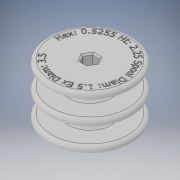
# Autodesk Inventor part: spool
Saved by Autodesk Inventor 2019.3 (Build 233278000, 278)
## iProperties
Created: 2019-02-25
Part Number: spool
Material: Generic
Document SubType Name: Modeling
Designer: steele
Density: 1 g/cm^3
Appearance: Default
Author: steele
Autodesk Inventor part; units mm, degrees
(part 1 of 2)
ref_plane "YZ Plane" through (0, 0, 0) normal (1, 0, 0) x (0, 1, 0)
ref_plane "XZ Plane" through (0, 0, 0) normal (0, 1, 0) x (-1, 0, 0)
ref_plane "XY Plane" through (0, 0, 0) normal (0, 0, 1) x (1, 0, 0)
sketch "Sketch1" plane through (0, 0, 0) normal (1, 0, 0) x (0, 1, 0)
  line L0 (0, 0) -> (0, -40.64)
  line L1 (3.81, -44.45) -> (3.81, -44.45)
  line L2 (7.62, -40.64) -> (7.62, -22.86)
  line L3 (11.43, -19.05) -> (20.955, -19.05)
  line L4 (24.765, -22.86) -> (24.765, -40.64)
  line L5 (28.575, -44.45) -> (28.575, -44.45)
  line L6 (32.385, -40.64) -> (32.385, -22.86)
  line L7 (36.195, -19.05) -> (45.72, -19.05)
  line L8 (49.53, -22.86) -> (49.53, -40.64)
  line L9 (53.34, -44.45) -> (53.34, -44.45)
  line L10 (57.15, -40.64) -> (57.15, 0)
  line L11 (0, 0) -> (57.15, 0)
  arc A0 (53.34, -44.45) -> (57.15, -40.64) centre (53.34, -40.64) ccw
  arc A1 (49.53, -40.64) -> (53.34, -44.45) centre (53.34, -40.64) ccw
  arc A2 (28.575, -44.45) -> (32.385, -40.64) centre (28.575, -40.64) ccw
  arc A3 (24.765, -40.64) -> (28.575, -44.45) centre (28.575, -40.64) ccw
  arc A4 (3.81, -44.45) -> (7.62, -40.64) centre (3.81, -40.64) ccw
  arc A5 (0, -40.64) -> (3.81, -44.45) centre (3.81, -40.64) ccw
  arc A6 (49.53, -22.86) -> (45.72, -19.05) centre (45.72, -22.86) ccw
  arc A7 (36.195, -19.05) -> (32.385, -22.86) centre (36.195, -22.86) ccw
  arc A8 (24.765, -22.86) -> (20.955, -19.05) centre (20.955, -22.86) ccw
  arc A9 (11.43, -19.05) -> (7.62, -22.86) centre (11.43, -22.86) ccw
  point P0 (49.53, -44.45)
  point P1 (57.15, -44.45)
  dimension "d0" = 57.15
  dimension "d1" = 7.62
  dimension "d2" = 19.05
  dimension "d3" = 44.45
  dimension "d4" = 3.81
  dimension "d5" = 3.81
  constraints: 24 end point, 20 point on circle, 20 tangent, 10 centre point, 8 equal radius, 6 perpendicular, 6 point on line, 5 collinear, 1 horizontal, 1 parallel, 1 vertical
  measures "d0" distance between parallel lines of L10 L0
  measures "d1" distance of point (49.53, -44.45) point (57.15, -44.45)
  measures "d2" distance between parallel lines of L3 L11
  measures "d3" distance between parallel lines of L1 L11
  measures "d4" radius of A0
  measures "d5" radius of A6
revolve "Revolution1" add sketch "Sketch1" angle 360 about axis through (0, 0, 0) along (0, 1, 0)
sketch "Sketch2" plane through (0, 57.15, 0) normal (0, 1, 0) x (1, 0, 0)
  line L0 (7.6623, 0) -> (3.8312, -6.6357)
  line L1 (3.8312, -6.6357) -> (-3.8312, -6.6357)
  line L2 (-3.8312, -6.6357) -> (-7.6623, 0)
  line L3 (-7.6623, 0) -> (-3.8312, 6.6357)
  line L4 (-3.8312, 6.6357) -> (3.8312, 6.6358)
  line L5 (3.8312, 6.6358) -> (7.6623, 0)
  point P0 (0, 0)
  point P1 (0, 0)
  dimension "d8" = 13.2715
  constraints: 12 end point, 1 coincident, 1 horizontal, 13 other
  measures "d8" distance between parallel lines of L1 L4
extrude "Extrusion1" cut sketch "Sketch2" against normal through all
sketch "Sketch4" plane through (0, 0, 0) normal (1, 0, 0) x (0, 1, 0)
  circle A0 centre (40.9575, 8.3858) radius 1.75
  circle A1 centre (16.1925, 8.3858) radius 1.75
  line L0 (7.62, 40.64) -> (7.62, -40.64) projected
  line L1 (49.53, 40.64) -> (49.53, -40.64) projected
  line L2 (57.15, 0) -> (0, 0) projected
  dimension "d17" = 8.5725
  dimension "d18" = 8.5725
  dimension "d19" = 3.5
  dimension "d20" = 8.3857
  dimension "d21" = 8.3857
  constraints: 2 centre point, 1 equal radius
  measures "d17" distance from line of A1.centre L0
  measures "d18" distance from line of A0.centre L1
  measures "d19" diameter of A0
  measures "d20" distance from line of A1.centre L2
  measures "d21" distance from line of A0.centre L2
extrude "Extrusion3" cut sketch "Sketch4" along normal through all both and the other way through all
chamfer "Chamfer2" distance 1.5875 angle 45 12 edges at (-5.7467, 57.15, -3.3179) (-5.7467, 57.15, 3.3179) (0, 57.15, 6.6357) (5.7467, 57.15, 3.3179) (0, 57.15, -6.6358) (0, 0, 6.6357) (5.7467, 0, 3.3179) (5.7467, 0, -3.3179) (0, 0, -6.6358) (-5.7467, 0, -3.3179) (-5.7467, 0, 3.3179) (5.7467, 57.15, -3.3179)
sketch "Sketch5" plane through (0, 57.15, 0) normal (0, 1, 0) x (1, 0, 0)
  circle A0 centre (0, 0) radius 33.3375
  line L0 (-33.0307, 5.0257) -> (-33.0993, 4.2184)
  line L1 (-33.0993, 4.2184) -> (-36.0724, 4.4709)
  line L2 (-36.0724, 4.4709) -> (-36.3098, 1.675)
  line L3 (-36.3098, 1.675) -> (-33.3367, 1.4226)
  line L4 (-33.3367, 1.4226) -> (-33.4052, 0.6153)
  line L5 (-33.4052, 0.6153) -> (-39.4794, 1.131)
  line L6 (-39.4794, 1.131) -> (-39.4108, 1.9383)
  line L7 (-39.4108, 1.9383) -> (-37.0284, 1.736)
  line L8 (-37.0284, 1.736) -> (-36.791, 4.5319)
  line L9 (-36.791, 4.5319) -> (-39.1734, 4.7342)
  line L10 (-39.1734, 4.7342) -> (-39.1049, 5.5414)
  line L11 (-39.1049, 5.5414) -> (-33.0307, 5.0257)
  spline S0 degree 2 poles (-32.2377, 8.0827) (-32.4935, 7.0163) (-33.9709, 6.1312) (-35.0757, 6.3963) knots 0 0 0 1 2 2 2
  spline S1 degree 2 poles (-35.0757, 6.3963) (-36.1614, 6.6568) (-37.1756, 8.1041) (-36.9555, 9.0216) knots 0 0 0 1 2 2 2
  spline S2 degree 2 poles (-36.9555, 9.0216) (-36.8563, 9.4348) (-36.4629, 10.016) (-36.1518, 10.1903) knots 0 0 0 1 2 2 2
  spline S3 degree 2 poles (-36.1518, 10.1903) (-35.8396, 10.3694) (-35.0435, 10.4477) (-34.5103, 10.3197) knots 0 0 0 1 2 2 2
  line L12 (-34.5103, 10.3197) -> (-34.102, 10.2218)
  line L13 (-34.102, 10.2218) -> (-34.8408, 7.1426)
  spline S4 degree 2 poles (-34.8408, 7.1426) (-34.0674, 6.957) (-33.0592, 7.5382) (-32.8933, 8.2299) knots 0 0 0 1 2 2 2
  spline S5 degree 2 poles (-32.8933, 8.2299) (-32.8345, 8.4749) (-32.8309, 8.9769) (-32.8712, 9.1898) knots 0 0 0 1 2 2 2
  spline S6 degree 2 poles (-32.8712, 9.1898) (-32.9189, 9.4147) (-33.0202, 9.7336) (-33.0751, 9.8433) knots 0 0 0 1 2 2 2
  line L14 (-33.0751, 9.8433) -> (-33.0648, 9.8865)
  line L15 (-33.0648, 9.8865) -> (-32.2481, 9.6906)
  spline S7 degree 2 poles (-32.2481, 9.6906) (-32.2264, 9.5482) (-32.1672, 9.1175) (-32.1609, 8.9534) knots 0 0 0 1 2 2 2
  spline S8 degree 2 poles (-32.1609, 8.9534) (-32.1503, 8.7222) (-32.1731, 8.3518) (-32.2377, 8.0827) knots 0 0 0 1 2 2 2
  spline S9 degree 2 poles (-34.8488, 9.6288) (-35.1538, 9.6918) (-35.6257, 9.6729) (-35.8034, 9.5885) knots 0 0 0 1 2 2 2
  spline S10 degree 2 poles (-35.8034, 9.5885) (-36.0026, 9.4992) (-36.2783, 9.1335) (-36.351, 8.8309) knots 0 0 0 1 2 2 2
  spline S11 degree 2 poles (-36.351, 8.8309) (-36.4224, 8.533) (-36.3449, 8.0725) (-36.2135, 7.8581) knots 0 0 0 1 2 2 2
  spline S12 degree 2 poles (-36.2135, 7.8581) (-36.0761, 7.6473) (-35.6901, 7.3718) (-35.4124, 7.2798) knots 0 0 0 1 2 2 2
  line L16 (-35.4124, 7.2798) -> (-34.8488, 9.6288)
  line L17 (-30.4327, 13.7615) -> (-30.7684, 12.8797)
  line L18 (-30.7684, 12.8797) -> (-32.7705, 12.4524)
  line L19 (-32.7705, 12.4524) -> (-31.5698, 10.7744)
  line L20 (-31.5698, 10.7744) -> (-31.8808, 9.9572)
  line L21 (-31.8808, 9.9572) -> (-33.4358, 12.2458)
  line L22 (-33.4358, 12.2458) -> (-36.1508, 11.5983)
  line L23 (-36.1508, 11.5983) -> (-35.8151, 12.4802)
  line L24 (-35.8151, 12.4802) -> (-33.8286, 12.9081)
  line L25 (-33.8286, 12.9081) -> (-35.019, 14.5716)
  line L26 (-35.019, 14.5716) -> (-34.708, 15.3888)
  line L27 (-34.708, 15.3888) -> (-33.1587, 13.1129)
  line L28 (-33.1587, 13.1129) -> (-30.4327, 13.7615)
  line L29 (-29.4968, 15.5425) -> (-29.94, 14.6706)
  line L30 (-29.94, 14.6706) -> (-30.9793, 15.1988)
  line L31 (-30.9793, 15.1988) -> (-30.536, 16.0708)
  line L32 (-30.536, 16.0708) -> (-29.4968, 15.5425)
  line L33 (-32.5353, 17.0871) -> (-32.9786, 16.2151)
  line L34 (-32.9786, 16.2151) -> (-34.0179, 16.7434)
  line L35 (-34.0179, 16.7434) -> (-33.5746, 17.6154)
  line L36 (-33.5746, 17.6154) -> (-32.5353, 17.0871)
  spline S13 degree 2 poles (-27.5071, 23.8971) (-26.2132, 22.8893) (-25.5869, 21.1931) (-26.1971, 20.4097) knots 0 0 0 1 2 2 2
  spline S14 degree 2 poles (-26.1971, 20.4097) (-26.8163, 19.6146) (-28.6316, 19.8324) (-29.8982, 20.819) knots 0 0 0 1 2 2 2
  spline S15 degree 2 poles (-29.8982, 20.819) (-31.2, 21.8328) (-31.8184, 23.523) (-31.2053, 24.3103) knots 0 0 0 1 2 2 2
  spline S16 degree 2 poles (-31.2053, 24.3103) (-30.5891, 25.1014) (-28.7621, 24.8745) (-27.5071, 23.8971) knots 0 0 0 1 2 2 2
  spline S17 degree 2 poles (-26.6852, 21.9295) (-26.8501, 22.2082) (-27.5221, 22.8568) (-28.0171, 23.2423) knots 0 0 0 1 2 2 2
  spline S18 degree 2 poles (-28.0171, 23.2423) (-28.5121, 23.6278) (-29.3016, 24.1175) (-29.623, 24.2113) knots 0 0 0 1 2 2 2
  spline S19 degree 2 poles (-29.623, 24.2113) (-29.9444, 24.3051) (-30.4619, 24.1633) (-30.6713, 23.8944) knots 0 0 0 1 2 2 2
  spline S20 degree 2 poles (-30.6713, 23.8944) (-30.8808, 23.6255) (-30.8976, 23.0813) (-30.7232, 22.7827) knots 0 0 0 1 2 2 2
  spline S21 degree 2 poles (-30.7232, 22.7827) (-30.5535, 22.494) (-29.8599, 21.841) (-29.3883, 21.4737) knots 0 0 0 1 2 2 2
  spline S22 degree 2 poles (-29.3883, 21.4737) (-28.8816, 21.0791) (-28.1549, 20.6133) (-27.8109, 20.5082) knots 0 0 0 1 2 2 2
  spline S23 degree 2 poles (-27.8109, 20.5082) (-27.4887, 20.4075) (-26.9496, 20.5449) (-26.731, 20.8255) knots 0 0 0 1 2 2 2
  spline S24 degree 2 poles (-26.731, 20.8255) (-26.5246, 21.0906) (-26.5078, 21.6347) (-26.6852, 21.9295) knots 0 0 0 1 2 2 2
  line L37 (-23.637, 23.5142) -> (-24.3167, 22.8108)
  line L38 (-24.3167, 22.8108) -> (-25.1551, 23.6209)
  line L39 (-25.1551, 23.6209) -> (-24.4754, 24.3243)
  line L40 (-24.4754, 24.3243) -> (-23.637, 23.5142)
  spline S25 degree 2 poles (-21.1932, 28.2583) (-20.9113, 27.9209) (-20.646, 27.1641) (-20.6658, 26.7871) knots 0 0 0 1 2 2 2
  spline S26 degree 2 poles (-20.6658, 26.7871) (-20.6856, 26.4101) (-21.0674, 25.6728) (-21.4313, 25.3688) knots 0 0 0 1 2 2 2
  spline S27 degree 2 poles (-21.4313, 25.3688) (-21.7649, 25.09) (-22.5405, 24.6932) (-22.8776, 24.6111) knots 0 0 0 1 2 2 2
  line L41 (-22.8776, 24.6111) -> (-23.4318, 25.2746)
  line L42 (-23.4318, 25.2746) -> (-23.3863, 25.3126)
  spline S28 degree 2 poles (-23.3863, 25.3126) (-23.2699, 25.3197) (-22.8868, 25.4081) (-22.6731, 25.4836) knots 0 0 0 1 2 2 2
  spline S29 degree 2 poles (-22.6731, 25.4836) (-22.4335, 25.5744) (-22.0662, 25.7589) (-21.8728, 25.9204) knots 0 0 0 1 2 2 2
  spline S30 degree 2 poles (-21.8728, 25.9204) (-21.6833, 26.0788) (-21.4409, 26.513) (-21.4356, 26.7685) knots 0 0 0 1 2 2 2
  spline S31 degree 2 poles (-21.4356, 26.7685) (-21.4352, 27.0069) (-21.6243, 27.4798) (-21.8333, 27.73) knots 0 0 0 1 2 2 2
  spline S32 degree 2 poles (-21.8333, 27.73) (-22.0423, 27.9803) (-22.4449, 28.1847) (-22.6624, 28.1832) knots 0 0 0 1 2 2 2
  spline S33 degree 2 poles (-22.6624, 28.1832) (-22.8933, 28.1899) (-23.3699, 27.959) (-23.6088, 27.7595) knots 0 0 0 1 2 2 2
  spline S34 degree 2 poles (-23.6088, 27.7595) (-23.8666, 27.5441) (-24.3119, 27.037) (-24.4388, 26.873) knots 0 0 0 1 2 2 2
  line L43 (-24.4388, 26.873) -> (-26.4531, 29.2842)
  line L44 (-26.4531, 29.2842) -> (-23.8865, 31.4283)
  line L45 (-23.8865, 31.4283) -> (-23.4273, 30.8786)
  line L46 (-23.4273, 30.8786) -> (-25.3911, 29.238)
  line L47 (-25.3911, 29.238) -> (-24.3491, 27.9907)
  spline S35 degree 2 poles (-24.3491, 27.9907) (-24.248, 28.1009) (-24.0377, 28.296) (-23.9467, 28.372) knots 0 0 0 1 2 2 2
  spline S36 degree 2 poles (-23.9467, 28.372) (-23.5865, 28.6729) (-22.9917, 28.9702) (-22.6185, 28.9859) knots 0 0 0 1 2 2 2
  spline S37 degree 2 poles (-22.6185, 28.9859) (-22.2416, 29.0047) (-21.5479, 28.683) (-21.1932, 28.2583) knots 0 0 0 1 2 2 2
  line L48 (-16.0539, 29.2803) -> (-19.2411, 27.2867)
  line L49 (-19.2411, 27.2867) -> (-19.6996, 28.0196)
  spline S38 degree 2 poles (-19.6996, 28.0196) (-19.5579, 28.5569) (-19.321, 29.5383) (-19.2295, 30.0442) knots 0 0 0 1 2 2 2
  spline S39 degree 2 poles (-19.2295, 30.0442) (-19.0451, 31.0627) (-19.1009, 32.1116) (-19.3603, 32.5262) knots 0 0 0 1 2 2 2
  spline S40 degree 2 poles (-19.3603, 32.5262) (-19.4965, 32.744) (-19.8349, 32.9868) (-20.0218, 33.0156) knots 0 0 0 1 2 2 2
  spline S41 degree 2 poles (-20.0218, 33.0156) (-20.2088, 33.0443) (-20.5926, 32.9499) (-20.7852, 32.8294) knots 0 0 0 1 2 2 2
  spline S42 degree 2 poles (-20.7852, 32.8294) (-20.9695, 32.7141) (-21.2888, 32.3862) (-21.416, 32.2076) knots 0 0 0 1 2 2 2
  spline S43 degree 2 poles (-21.416, 32.2076) (-21.5259, 32.0573) (-21.6934, 31.7195) (-21.7404, 31.6085) knots 0 0 0 1 2 2 2
  line L50 (-21.7404, 31.6085) -> (-21.7781, 31.5849)
  line L51 (-21.7781, 31.5849) -> (-22.2392, 32.322)
  spline S44 degree 2 poles (-22.2392, 32.322) (-22.0911, 32.5603) (-21.453, 33.2449) (-21.1096, 33.4598) knots 0 0 0 1 2 2 2
  spline S45 degree 2 poles (-21.1096, 33.4598) (-20.385, 33.913) (-19.0889, 33.6574) (-18.6803, 33.004) knots 0 0 0 1 2 2 2
  spline S46 degree 2 poles (-18.6803, 33.004) (-18.489, 32.6983) (-18.3118, 32.0982) (-18.3012, 31.8019) knots 0 0 0 1 2 2 2
  spline S47 degree 2 poles (-18.3012, 31.8019) (-18.2854, 31.4971) (-18.3721, 30.8252) (-18.4395, 30.4859) knots 0 0 0 1 2 2 2
  spline S48 degree 2 poles (-18.4395, 30.4859) (-18.5435, 29.9256) (-18.8667, 28.6629) (-18.9666, 28.2916) knots 0 0 0 1 2 2 2
  line L52 (-18.9666, 28.2916) -> (-16.4285, 29.8792)
  line L53 (-16.4285, 29.8792) -> (-16.0539, 29.2803)
  spline S49 degree 2 poles (-12.7562, 32.9388) (-12.5762, 32.5377) (-12.5255, 31.7374) (-12.6466, 31.3798) knots 0 0 0 1 2 2 2
  spline S50 degree 2 poles (-12.6466, 31.3798) (-12.7676, 31.0222) (-13.3347, 30.4157) (-13.7673, 30.2214) knots 0 0 0 1 2 2 2
  spline S51 degree 2 poles (-13.7673, 30.2214) (-14.1639, 30.0434) (-15.018, 29.8712) (-15.3646, 29.8834) knots 0 0 0 1 2 2 2
  line L54 (-15.3646, 29.8834) -> (-15.7187, 30.6721)
  line L55 (-15.7187, 30.6721) -> (-15.6646, 30.6964)
  spline S52 degree 2 poles (-15.6646, 30.6964) (-15.5506, 30.6717) (-15.1578, 30.6531) (-14.9317, 30.668) knots 0 0 0 1 2 2 2
  spline S53 degree 2 poles (-14.9317, 30.668) (-14.6764, 30.6906) (-14.273, 30.7688) (-14.0431, 30.872) knots 0 0 0 1 2 2 2
  spline S54 degree 2 poles (-14.0431, 30.872) (-13.8178, 30.9731) (-13.467, 31.3256) (-13.3926, 31.5701) knots 0 0 0 1 2 2 2
  spline S55 degree 2 poles (-13.3926, 31.5701) (-13.3278, 31.7996) (-13.3818, 32.306) (-13.5154, 32.6034) knots 0 0 0 1 2 2 2
  spline S56 degree 2 poles (-13.5154, 32.6034) (-13.6489, 32.9009) (-13.9811, 33.2066) (-14.191, 33.264) knots 0 0 0 1 2 2 2
  spline S57 degree 2 poles (-14.191, 33.264) (-14.4114, 33.3329) (-14.9327, 33.2397) (-15.2167, 33.1122) knots 0 0 0 1 2 2 2
  spline S58 degree 2 poles (-15.2167, 33.1122) (-15.5231, 32.9746) (-16.089, 32.6069) (-16.2556, 32.4834) knots 0 0 0 1 2 2 2
  line L56 (-16.2556, 32.4834) -> (-17.5423, 35.3496)
  line L57 (-17.5423, 35.3496) -> (-14.4913, 36.7193)
  line L58 (-14.4913, 36.7193) -> (-14.1979, 36.0658)
  line L59 (-14.1979, 36.0658) -> (-16.5324, 35.0179)
  line L60 (-16.5324, 35.0179) -> (-15.8668, 33.5351)
  spline S59 degree 2 poles (-15.8668, 33.5351) (-15.7397, 33.6139) (-15.4844, 33.7447) (-15.3762, 33.7933) knots 0 0 0 1 2 2 2
  spline S60 degree 2 poles (-15.3762, 33.7933) (-14.9481, 33.9855) (-14.2949, 34.1108) (-13.9315, 34.0249) knots 0 0 0 1 2 2 2
  spline S61 degree 2 poles (-13.9315, 34.0249) (-13.5635, 33.941) (-12.9828, 33.4436) (-12.7562, 32.9388) knots 0 0 0 1 2 2 2
  spline S62 degree 2 poles (-8.1381, 34.3723) (-8.0145, 33.9504) (-8.0737, 33.1506) (-8.2424, 32.8129) knots 0 0 0 1 2 2 2
  spline S63 degree 2 poles (-8.2424, 32.8129) (-8.4112, 32.4752) (-9.0557, 31.9518) (-9.5109, 31.8185) knots 0 0 0 1 2 2 2
  spline S64 degree 2 poles (-9.5109, 31.8185) (-9.928, 31.6963) (-10.7976, 31.6424) (-11.1393, 31.7018) knots 0 0 0 1 2 2 2
  line L61 (-11.1393, 31.7018) -> (-11.3824, 32.5315)
  line L62 (-11.3824, 32.5315) -> (-11.3255, 32.5481)
  spline S65 degree 2 poles (-11.3255, 32.5481) (-11.216, 32.5082) (-10.8294, 32.4361) (-10.6033, 32.4199) knots 0 0 0 1 2 2 2
  spline S66 degree 2 poles (-10.6033, 32.4199) (-10.3474, 32.4074) (-9.937, 32.4298) (-9.6952, 32.5006) knots 0 0 0 1 2 2 2
  spline S67 degree 2 poles (-9.6952, 32.5006) (-9.4582, 32.5701) (-9.0625, 32.8713) (-8.9555, 33.1034) knots 0 0 0 1 2 2 2
  spline S68 degree 2 poles (-8.9555, 33.1034) (-8.8599, 33.3218) (-8.8443, 33.8309) (-8.936, 34.1438) knots 0 0 0 1 2 2 2
  spline S69 degree 2 poles (-8.936, 34.1438) (-9.0276, 34.4567) (-9.3149, 34.8049) (-9.515, 34.8904) knots 0 0 0 1 2 2 2
  spline S70 degree 2 poles (-9.515, 34.8904) (-9.724, 34.9888) (-10.2531, 34.9676) (-10.5518, 34.8801) knots 0 0 0 1 2 2 2
  spline S71 degree 2 poles (-10.5518, 34.8801) (-10.8742, 34.7857) (-11.485, 34.4987) (-11.6669, 34.3991) knots 0 0 0 1 2 2 2
  line L63 (-11.6669, 34.3991) -> (-12.5501, 37.4142)
  line L64 (-12.5501, 37.4142) -> (-9.3406, 38.3544)
  line L65 (-9.3406, 38.3544) -> (-9.1392, 37.667)
  line L66 (-9.1392, 37.667) -> (-11.595, 36.9476)
  line L67 (-11.595, 36.9476) -> (-11.1381, 35.3879)
  spline S72 degree 2 poles (-11.1381, 35.3879) (-11.0014, 35.4485) (-10.7306, 35.5433) (-10.6168, 35.5766) knots 0 0 0 1 2 2 2
  spline S73 degree 2 poles (-10.6168, 35.5766) (-10.1665, 35.7085) (-9.5024, 35.7435) (-9.154, 35.6087) knots 0 0 0 1 2 2 2
  spline S74 degree 2 poles (-9.154, 35.6087) (-8.801, 35.4754) (-8.2936, 34.9033) (-8.1381, 34.3723) knots 0 0 0 1 2 2 2
  line L68 (0.4356, 33.408) -> (-0.3734, 33.3649)
  line L69 (-0.3734, 33.3649) -> (-0.5322, 36.3445)
  line L70 (-0.5322, 36.3445) -> (-3.3341, 36.1951)
  line L71 (-3.3341, 36.1951) -> (-3.1753, 33.2156)
  line L72 (-3.1753, 33.2156) -> (-3.9843, 33.1725)
  line L73 (-3.9843, 33.1725) -> (-4.3088, 39.2598)
  line L74 (-4.3088, 39.2598) -> (-3.4998, 39.3029)
  line L75 (-3.4998, 39.3029) -> (-3.3725, 36.9153)
  line L76 (-3.3725, 36.9153) -> (-0.5706, 37.0647)
  line L77 (-0.5706, 37.0647) -> (-0.6978, 39.4523)
  line L78 (-0.6978, 39.4523) -> (0.1112, 39.4954)
  line L79 (0.1112, 39.4954) -> (0.4356, 33.408)
  spline S75 degree 2 poles (2.9791, 33.1192) (2.3534, 33.1653) (1.7015, 33.9316) (1.7585, 34.7051) knots 0 0 0 1 2 2 2
  line L80 (1.7585, 34.7051) -> (1.9446, 37.2324)
  line L81 (1.9446, 37.2324) -> (1.4273, 37.2705)
  line L82 (1.4273, 37.2705) -> (1.4741, 37.9061)
  line L83 (1.4741, 37.9061) -> (1.9914, 37.868)
  line L84 (1.9914, 37.868) -> (2.0879, 39.1785)
  line L85 (2.0879, 39.1785) -> (2.8565, 39.1219)
  line L86 (2.8565, 39.1219) -> (2.76, 37.8114)
  line L87 (2.76, 37.8114) -> (4.1739, 37.7072)
  line L88 (4.1739, 37.7072) -> (4.1271, 37.0717)
  line L89 (4.1271, 37.0717) -> (2.7132, 37.1758)
  line L90 (2.7132, 37.1758) -> (2.5532, 35.0032)
  spline S76 degree 2 poles (2.5532, 35.0032) (2.5278, 34.6583) (2.5244, 34.2771) (2.5962, 34.1084) knots 0 0 0 1 2 2 2
  spline S77 degree 2 poles (2.5962, 34.1084) (2.6547, 33.9604) (2.9545, 33.7947) (3.2206, 33.7751) knots 0 0 0 1 2 2 2
  spline S78 degree 2 poles (3.2206, 33.7751) (3.4078, 33.7613) (3.7659, 33.8489) (3.8473, 33.8775) knots 0 0 0 1 2 2 2
  line L91 (3.8473, 33.8775) -> (3.8916, 33.8743)
  line L92 (3.8916, 33.8743) -> (3.8408, 33.1845)
  spline S79 degree 2 poles (3.8408, 33.1845) (3.6197, 33.1414) (3.1712, 33.1051) (2.9791, 33.1192) knots 0 0 0 1 2 2 2
  line L93 (6.3371, 36.1989) -> (5.3715, 36.3547)
  line L94 (5.3715, 36.3547) -> (5.5572, 37.5056)
  line L95 (5.5572, 37.5056) -> (6.5229, 37.3498)
  line L96 (6.5229, 37.3498) -> (6.3371, 36.1989)
  line L97 (5.7941, 32.8338) -> (4.8284, 32.9896)
  line L98 (4.8284, 32.9896) -> (5.0142, 34.1406)
  line L99 (5.0142, 34.1406) -> (5.9798, 33.9847)
  line L100 (5.9798, 33.9847) -> (5.7941, 32.8338)
  line L101 (13.2755, 30.6402) -> (9.7459, 31.9343)
  line L102 (9.7459, 31.9343) -> (10.0435, 32.746)
  spline S80 degree 2 poles (10.0435, 32.746) (10.5547, 32.9637) (11.4751, 33.3787) (11.9307, 33.6168) knots 0 0 0 1 2 2 2
  spline S81 degree 2 poles (11.9307, 33.6168) (12.8482, 34.0959) (13.6423, 34.7834) (13.8106, 35.2426) knots 0 0 0 1 2 2 2
  spline S82 degree 2 poles (13.8106, 35.2426) (13.8991, 35.4838) (13.8833, 35.9) (13.7913, 36.0653) knots 0 0 0 1 2 2 2
  spline S83 degree 2 poles (13.7913, 36.0653) (13.6993, 36.2305) (13.3893, 36.4757) (13.176, 36.5539) knots 0 0 0 1 2 2 2
  spline S84 degree 2 poles (13.176, 36.5539) (12.9719, 36.6288) (12.517, 36.6798) (12.298, 36.6706) knots 0 0 0 1 2 2 2
  spline S85 degree 2 poles (12.298, 36.6706) (12.1118, 36.6652) (11.7423, 36.5902) (11.6258, 36.5593) knots 0 0 0 1 2 2 2
  line L103 (11.6258, 36.5593) -> (11.584, 36.5746)
  line L104 (11.584, 36.5746) -> (11.8833, 37.3909)
  spline S86 degree 2 poles (11.8833, 37.3909) (12.1624, 37.4202) (13.0945, 37.3362) (13.4748, 37.1968) knots 0 0 0 1 2 2 2
  spline S87 degree 2 poles (13.4748, 37.1968) (14.2772, 36.9026) (14.8704, 35.7222) (14.6051, 34.9987) knots 0 0 0 1 2 2 2
  spline S88 degree 2 poles (14.6051, 34.9987) (14.481, 34.6601) (14.1158, 34.1521) (13.8883, 33.9619) knots 0 0 0 1 2 2 2
  spline S89 degree 2 poles (13.8883, 33.9619) (13.6573, 33.7624) (13.0735, 33.4188) (12.7642, 33.2638) knots 0 0 0 1 2 2 2
  spline S90 degree 2 poles (12.7642, 33.2638) (12.2578, 33.0022) (11.0625, 32.4829) (10.708, 32.334) knots 0 0 0 1 2 2 2
  line L105 (10.708, 32.334) -> (13.5187, 31.3035)
  line L106 (13.5187, 31.3035) -> (13.2755, 30.6402)
  line L107 (15.1742, 29.6878) -> (14.2969, 30.1203)
  line L108 (14.2969, 30.1203) -> (14.8124, 31.166)
  line L109 (14.8124, 31.166) -> (15.6897, 30.7335)
  line L110 (15.6897, 30.7335) -> (15.1742, 29.6878)
  line L111 (19.4562, 27.1389) -> (16.2802, 29.1503)
  line L112 (16.2802, 29.1503) -> (16.7427, 29.8807)
  spline S91 degree 2 poles (16.7427, 29.8807) (17.2885, 29.9853) (18.2757, 30.1962) (18.7714, 30.3325) knots 0 0 0 1 2 2 2
  spline S92 degree 2 poles (18.7714, 30.3325) (19.7695, 30.6068) (20.691, 31.1108) (20.9527, 31.524) knots 0 0 0 1 2 2 2
  spline S93 degree 2 poles (20.9527, 31.524) (21.0901, 31.741) (21.1628, 32.1511) (21.1078, 32.3321) knots 0 0 0 1 2 2 2
  spline S94 degree 2 poles (21.1078, 32.3321) (21.0528, 32.5131) (20.8017, 32.8183) (20.6098, 32.9399) knots 0 0 0 1 2 2 2
  spline S95 degree 2 poles (20.6098, 32.9399) (20.4261, 33.0562) (19.9924, 33.2022) (19.7763, 33.2396) knots 0 0 0 1 2 2 2
  spline S96 degree 2 poles (19.7763, 33.2396) (19.5932, 33.2737) (19.2162, 33.2786) (19.0958, 33.273) knots 0 0 0 1 2 2 2
  line L113 (19.0958, 33.273) -> (19.0582, 33.2968)
  line L114 (19.0582, 33.2968) -> (19.5234, 34.0313)
  spline S97 degree 2 poles (19.5234, 34.0313) (19.8023, 34.0009) (20.6956, 33.7217) (21.0378, 33.5049) knots 0 0 0 1 2 2 2
  spline S98 degree 2 poles (21.0378, 33.5049) (21.7598, 33.0477) (22.09, 31.7685) (21.6776, 31.1175) knots 0 0 0 1 2 2 2
  spline S99 degree 2 poles (21.6776, 31.1175) (21.4847, 30.8128) (21.0203, 30.3935) (20.7577, 30.2558) knots 0 0 0 1 2 2 2
  spline S100 degree 2 poles (20.7577, 30.2558) (20.4898, 30.1097) (19.8465, 29.8973) (19.5114, 29.8113) knots 0 0 0 1 2 2 2
  spline S101 degree 2 poles (19.5114, 29.8113) (18.9612, 29.6627) (17.683, 29.408) (17.305, 29.3374) knots 0 0 0 1 2 2 2
  line L115 (17.305, 29.3374) -> (19.8341, 27.7357)
  line L116 (19.8341, 27.7357) -> (19.4562, 27.1389)
  spline S102 degree 2 poles (24.1811, 25.748) (23.8973, 25.4122) (23.1976, 25.0204) (22.8229, 24.9748) knots 0 0 0 1 2 2 2
  spline S103 degree 2 poles (22.8229, 24.9748) (22.4481, 24.9293) (21.656, 25.1783) (21.2938, 25.4843) knots 0 0 0 1 2 2 2
  spline S104 degree 2 poles (21.2938, 25.4843) (20.9617, 25.7649) (20.437, 26.4605) (20.2981, 26.7783) knots 0 0 0 1 2 2 2
  line L117 (20.2981, 26.7783) -> (20.8561, 27.4386)
  line L118 (20.8561, 27.4386) -> (20.9014, 27.4004)
  spline S105 degree 2 poles (20.9014, 27.4004) (20.9284, 27.287) (21.0816, 26.9248) (21.1928, 26.7273) knots 0 0 0 1 2 2 2
  spline S106 degree 2 poles (21.1928, 26.7273) (21.3235, 26.5069) (21.5686, 26.177) (21.761, 26.0144) knots 0 0 0 1 2 2 2
  spline S107 degree 2 poles (21.761, 26.0144) (21.9497, 25.8549) (22.4192, 25.6911) (22.6718, 25.7298) knots 0 0 0 1 2 2 2
  spline S108 degree 2 poles (22.6718, 25.7298) (22.9067, 25.7706) (23.3399, 26.0384) (23.5504, 26.2874) knots 0 0 0 1 2 2 2
  spline S109 degree 2 poles (23.5504, 26.2874) (23.7608, 26.5365) (23.8928, 26.9682) (23.8538, 27.1823) knots 0 0 0 1 2 2 2
  spline S110 degree 2 poles (23.8538, 27.1823) (23.8205, 27.4108) (23.511, 27.8405) (23.2733, 28.0414) knots 0 0 0 1 2 2 2
  spline S111 degree 2 poles (23.2733, 28.0414) (23.0167, 28.2582) (22.4403, 28.6094) (22.2569, 28.7062) knots 0 0 0 1 2 2 2
  line L119 (22.2569, 28.7062) -> (24.2847, 31.106)
  line L120 (24.2847, 31.106) -> (26.8393, 28.9475)
  line L121 (26.8393, 28.9475) -> (26.377, 28.4004)
  line L122 (26.377, 28.4004) -> (24.4224, 30.0519)
  line L123 (24.4224, 30.0519) -> (23.3734, 28.8105)
  spline S112 degree 2 poles (23.3734, 28.8105) (23.4993, 28.7299) (23.7278, 28.5563) (23.8183, 28.4798) knots 0 0 0 1 2 2 2
  spline S113 degree 2 poles (23.8183, 28.4798) (24.1768, 28.1769) (24.5723, 27.6423) (24.652, 27.2774) knots 0 0 0 1 2 2 2
  spline S114 degree 2 poles (24.652, 27.2774) (24.7355, 26.9093) (24.5382, 26.1706) (24.1811, 25.748) knots 0 0 0 1 2 2 2
  spline S115 degree 2 poles (26.3953, 20.1852) (25.9934, 20.7113) (25.6495, 21.6172) (25.5576, 22.063) knots 0 0 0 1 2 2 2
  line L124 (25.5576, 22.063) -> (26.3663, 22.6808)
  line L125 (26.3663, 22.6808) -> (26.4023, 22.6337)
  spline S116 degree 2 poles (26.4023, 22.6337) (26.3469, 22.0878) (26.6319, 21.0311) (26.9168, 20.6582) knots 0 0 0 1 2 2 2
  spline S117 degree 2 poles (26.9168, 20.6582) (27.3246, 20.1243) (28.185, 19.9175) (28.5501, 20.1964) knots 0 0 0 1 2 2 2
  spline S118 degree 2 poles (28.5501, 20.1964) (28.8406, 20.4183) (28.9829, 20.9807) (28.8362, 21.3598) knots 0 0 0 1 2 2 2
  spline S119 degree 2 poles (28.8362, 21.3598) (28.7281, 21.6316) (28.5296, 22.0705) (28.3873, 22.4032) knots 0 0 0 1 2 2 2
  spline S120 degree 2 poles (28.3873, 22.4032) (28.2622, 22.7054) (28.1595, 23.2549) (28.2035, 23.5309) knots 0 0 0 1 2 2 2
  spline S121 degree 2 poles (28.2035, 23.5309) (28.2505, 23.803) (28.5564, 24.2978) (28.839, 24.5137) knots 0 0 0 1 2 2 2
  spline S122 degree 2 poles (28.839, 24.5137) (29.4279, 24.9635) (30.9265, 24.6537) (31.4693, 23.9431) knots 0 0 0 1 2 2 2
  spline S123 degree 2 poles (31.4693, 23.9431) (31.7812, 23.5349) (32.172, 22.6896) (32.2558, 22.2625) knots 0 0 0 1 2 2 2
  line L126 (32.2558, 22.2625) -> (31.4864, 21.6747)
  line L127 (31.4864, 21.6747) -> (31.4504, 21.7219)
  spline S124 degree 2 poles (31.4504, 21.7219) (31.4854, 22.1154) (31.2477, 23.0776) (30.9448, 23.4741) knots 0 0 0 1 2 2 2
  spline S125 degree 2 poles (30.9448, 23.4741) (30.603, 23.9217) (29.7601, 24.1543) (29.4185, 23.8934) knots 0 0 0 1 2 2 2
  spline S126 degree 2 poles (29.4185, 23.8934) (29.1123, 23.6595) (28.9962, 23.0548) (29.1476, 22.6856) knots 0 0 0 1 2 2 2
  spline S127 degree 2 poles (29.1476, 22.6856) (29.2486, 22.4395) (29.5601, 21.7387) (29.6512, 21.4975) knots 0 0 0 1 2 2 2
  spline S128 degree 2 poles (29.6512, 21.4975) (29.8789, 20.882) (29.6164, 19.9479) (29.165, 19.603) knots 0 0 0 1 2 2 2
  spline S129 degree 2 poles (29.165, 19.603) (28.8784, 19.3841) (28.1519, 19.1959) (27.8006, 19.257) knots 0 0 0 1 2 2 2
  spline S130 degree 2 poles (27.8006, 19.257) (27.4117, 19.3267) (26.7342, 19.7416) (26.3953, 20.1852) knots 0 0 0 1 2 2 2
  spline S131 degree 2 poles (32.1641, 15.7389) (31.1655, 15.1764) (29.4504, 15.4632) (29.0406, 16.1906) knots 0 0 0 1 2 2 2
  spline S132 degree 2 poles (29.0406, 16.1906) (28.8733, 16.4875) (28.754, 17.0214) (28.7626, 17.3381) knots 0 0 0 1 2 2 2
  line L128 (28.7626, 17.3381) -> (27.0927, 16.3973)
  line L129 (27.0927, 16.3973) -> (26.7144, 17.0687)
  line L130 (26.7144, 17.0687) -> (32.1676, 20.1409)
  line L131 (32.1676, 20.1409) -> (32.5459, 19.4695)
  line L132 (32.5459, 19.4695) -> (32.1284, 19.2343)
  spline S133 degree 2 poles (32.1284, 19.2343) (32.4971, 19.1131) (33.1427, 18.6717) (33.344, 18.3145) knots 0 0 0 1 2 2 2
  spline S134 degree 2 poles (33.344, 18.3145) (33.7295, 17.6301) (33.0765, 16.253) (32.1641, 15.7389) knots 0 0 0 1 2 2 2
  spline S135 degree 2 poles (31.6962, 16.3882) (32.3805, 16.7738) (32.8888, 17.6328) (32.6148, 18.1192) knots 0 0 0 1 2 2 2
  spline S136 degree 2 poles (32.6148, 18.1192) (32.4548, 18.4032) (31.9002, 18.7939) (31.5689, 18.919) knots 0 0 0 1 2 2 2
  line L133 (31.5689, 18.919) -> (29.305, 17.6436)
  spline S137 degree 2 poles (29.305, 17.6436) (29.328, 17.3108) (29.4443, 16.883) (29.5801, 16.6419) knots 0 0 0 1 2 2 2
  spline S138 degree 2 poles (29.5801, 16.6419) (29.8735, 16.1212) (30.9645, 15.976) (31.6962, 16.3882) knots 0 0 0 1 2 2 2
  spline S139 degree 2 poles (33.8913, 11.1657) (32.8159, 10.7417) (31.2363, 11.3138) (30.8957, 12.1778) knots 0 0 0 1 2 2 2
  spline S140 degree 2 poles (30.8957, 12.1778) (30.546, 13.0647) (31.3543, 14.5569) (32.3929, 14.9664) knots 0 0 0 1 2 2 2
  spline S141 degree 2 poles (32.3929, 14.9664) (33.4591, 15.3868) (35.0534, 14.8046) (35.3904, 13.9498) knots 0 0 0 1 2 2 2
  spline S142 degree 2 poles (35.3904, 13.9498) (35.731, 13.0857) (34.9621, 11.5879) (33.8913, 11.1657) knots 0 0 0 1 2 2 2
  spline S143 degree 2 poles (33.5996, 11.9056) (34.4268, 12.2318) (34.9938, 13.1509) (34.7745, 13.707) knots 0 0 0 1 2 2 2
  spline S144 degree 2 poles (34.7745, 13.707) (34.5553, 14.2631) (33.5119, 14.5526) (32.6846, 14.2265) knots 0 0 0 1 2 2 2
  spline S145 degree 2 poles (32.6846, 14.2265) (31.8804, 13.9094) (31.2923, 12.9766) (31.5115, 12.4206) knots 0 0 0 1 2 2 2
  spline S146 degree 2 poles (31.5115, 12.4206) (31.7289, 11.8691) (32.7816, 11.5831) (33.5996, 11.9056) knots 0 0 0 1 2 2 2
  spline S147 degree 2 poles (35.0939, 6.4583) (33.9709, 6.1843) (32.4837, 6.9656) (32.2636, 7.8679) knots 0 0 0 1 2 2 2
  spline S148 degree 2 poles (32.2636, 7.8679) (32.0376, 8.7942) (33.0411, 10.1627) (34.1257, 10.4273) knots 0 0 0 1 2 2 2
  spline S149 degree 2 poles (34.1257, 10.4273) (35.2392, 10.6989) (36.7395, 9.9056) (36.9573, 9.0129) knots 0 0 0 1 2 2 2
  spline S150 degree 2 poles (36.9573, 9.0129) (37.1774, 8.1106) (36.2122, 6.7311) (35.0939, 6.4583) knots 0 0 0 1 2 2 2
  spline S151 degree 2 poles (34.9055, 7.231) (35.7693, 7.4417) (36.4558, 8.2753) (36.3142, 8.856) knots 0 0 0 1 2 2 2
  spline S152 degree 2 poles (36.3142, 8.856) (36.1725, 9.4367) (35.1781, 9.8654) (34.3142, 9.6546) knots 0 0 0 1 2 2 2
  spline S153 degree 2 poles (34.3142, 9.6546) (33.4743, 9.4497) (32.765, 8.6055) (32.9067, 8.0248) knots 0 0 0 1 2 2 2
  spline S154 degree 2 poles (32.9067, 8.0248) (33.0472, 7.4489) (34.0512, 7.0226) (34.9055, 7.231) knots 0 0 0 1 2 2 2
  line L134 (33.0548, 4.3497) -> (32.9454, 5.1126)
  line L135 (32.9454, 5.1126) -> (39.2486, 6.0162)
  line L136 (39.2486, 6.0162) -> (39.358, 5.2534)
  line L137 (39.358, 5.2534) -> (33.0548, 4.3497)
  spline S155 degree 2 poles (36.2065, -4.393) (35.3727, -4.3514) (34.0644, -3.6084) (33.7178, -3.0223) knots 0 0 0 1 2 2 2
  spline S156 degree 2 poles (33.7178, -3.0223) (33.4498, -2.5439) (33.3001, -1.5818) (33.337, -0.8418) knots 0 0 0 1 2 2 2
  line L138 (33.337, -0.8418) -> (33.407, 0.5595)
  line L139 (33.407, 0.5595) -> (39.4954, 0.2553)
  line L140 (39.4954, 0.2553) -> (39.4262, -1.1311)
  spline S157 degree 2 poles (39.4262, -1.1311) (39.3833, -1.9896) (39.0779, -2.9537) (38.8337, -3.2877) knots 0 0 0 1 2 2 2
  spline S158 degree 2 poles (38.8337, -3.2877) (38.4146, -3.8554) (37.0946, -4.4374) (36.2065, -4.393) knots 0 0 0 1 2 2 2
  spline S159 degree 2 poles (36.2585, -3.5498) (36.9591, -3.5848) (37.974, -3.1706) (38.2781, -2.7258) knots 0 0 0 1 2 2 2
  spline S160 degree 2 poles (38.2781, -2.7258) (38.4868, -2.4097) (38.6962, -1.6832) (38.7236, -1.1356) knots 0 0 0 1 2 2 2
  line L141 (38.7236, -1.1356) -> (38.7544, -0.5188)
  line L142 (38.7544, -0.5188) -> (34.0672, -0.2847)
  line L143 (34.0672, -0.2847) -> (34.0364, -0.9014)
  spline S161 degree 2 poles (34.0364, -0.9014) (34.0095, -1.4392) (34.1416, -2.2619) (34.3569, -2.6041) knots 0 0 0 1 2 2 2
  spline S162 degree 2 poles (34.3569, -2.6041) (34.6219, -3.0427) (35.548, -3.5143) (36.2585, -3.5498) knots 0 0 0 1 2 2 2
  line L144 (32.8289, -5.814) -> (32.9545, -5.0536)
  line L145 (32.9545, -5.0536) -> (37.4678, -5.7993)
  line L146 (37.4678, -5.7993) -> (37.3422, -6.5596)
  line L147 (37.3422, -6.5596) -> (32.8289, -5.814)
  line L148 (38.0839, -6.7372) -> (38.2264, -5.8745)
  line L149 (38.2264, -5.8745) -> (39.016, -6.005)
  line L150 (39.016, -6.005) -> (38.8735, -6.8676)
  line L151 (38.8735, -6.8676) -> (38.0839, -6.7372)
  spline S163 degree 2 poles (32.4673, -9.5184) (32.4244, -9.41) (32.2664, -9.0412) (32.2326, -8.879) knots 0 0 0 1 2 2 2
  spline S164 degree 2 poles (32.2326, -8.879) (32.1793, -8.6554) (32.1666, -8.2587) (32.255, -7.9243) knots 0 0 0 1 2 2 2
  spline S165 degree 2 poles (32.255, -7.9243) (32.3269, -7.6521) (32.6623, -7.2144) (32.8978, -7.0774) knots 0 0 0 1 2 2 2
  spline S166 degree 2 poles (32.8978, -7.0774) (33.126, -6.9487) (33.7177, -6.8751) (34.0138, -6.9534) knots 0 0 0 1 2 2 2
  spline S167 degree 2 poles (34.0138, -6.9534) (34.4723, -7.0745) (35.0196, -7.6331) (35.0948, -8.1026) knots 0 0 0 1 2 2 2
  spline S168 degree 2 poles (35.0948, -8.1026) (35.1683, -8.5206) (35.0296, -9.5672) (34.9078, -10.1635) knots 0 0 0 1 2 2 2
  line L152 (34.9078, -10.1635) -> (35.0511, -10.2013)
  spline S169 degree 2 poles (35.0511, -10.2013) (35.309, -10.2695) (35.6707, -10.1965) (35.7993, -10.0772) knots 0 0 0 1 2 2 2
  spline S170 degree 2 poles (35.7993, -10.0772) (35.9279, -9.9579) (36.0938, -9.5623) (36.1518, -9.3426) knots 0 0 0 1 2 2 2
  spline S171 degree 2 poles (36.1518, -9.3426) (36.22, -9.0847) (36.2514, -8.347) (36.1955, -7.9592) knots 0 0 0 1 2 2 2
  line L153 (36.1955, -7.9592) -> (36.2069, -7.9162)
  line L154 (36.2069, -7.9162) -> (36.9663, -8.1169)
  spline S172 degree 2 poles (36.9663, -8.1169) (36.9693, -8.3374) (36.9094, -9.1442) (36.8096, -9.5215) knots 0 0 0 1 2 2 2
  spline S173 degree 2 poles (36.8096, -9.5215) (36.6885, -9.98) (36.3798, -10.5678) (36.1279, -10.767) knots 0 0 0 1 2 2 2
  spline S174 degree 2 poles (36.1279, -10.767) (35.8821, -10.9626) (35.241, -11.0486) (34.8255, -10.9388) knots 0 0 0 1 2 2 2
  line L155 (34.8255, -10.9388) -> (31.8023, -10.1398)
  line L156 (31.8023, -10.1398) -> (31.9992, -9.3947)
  line L157 (31.9992, -9.3947) -> (32.4673, -9.5184)
  line L158 (33.0881, -9.6825) -> (34.3156, -10.0069)
  spline S175 degree 2 poles (34.3156, -10.0069) (34.3624, -9.7332) (34.4945, -8.9046) (34.485, -8.6312) knots 0 0 0 1 2 2 2
  spline S176 degree 2 poles (34.485, -8.6312) (34.4725, -8.3111) (34.1975, -7.8246) (33.8631, -7.7362) knots 0 0 0 1 2 2 2
  spline S177 degree 2 poles (33.8631, -7.7362) (33.4811, -7.6352) (32.9806, -7.9628) (32.872, -8.3736) knots 0 0 0 1 2 2 2
  spline S178 degree 2 poles (32.872, -8.3736) (32.7799, -8.7222) (32.9293, -9.3749) (33.0881, -9.6825) knots 0 0 0 1 2 2 2
  line L159 (29.383, -15.9054) -> (31.7903, -17.008)
  spline S179 degree 2 poles (31.7903, -17.008) (32.0778, -17.1397) (32.5879, -17.319) (32.7556, -17.3088) knots 0 0 0 1 2 2 2
  spline S180 degree 2 poles (32.7556, -17.3088) (32.9367, -17.3049) (33.2059, -17.0967) (33.3149, -16.8587) knots 0 0 0 1 2 2 2
  spline S181 degree 2 poles (33.3149, -16.8587) (33.4137, -16.6431) (33.375, -16.0277) (33.2427, -15.652) knots 0 0 0 1 2 2 2
  spline S182 degree 2 poles (33.2427, -15.652) (33.1778, -15.6277) (32.9985, -15.5564) (32.8818, -15.5029) knots 0 0 0 1 2 2 2
  line L160 (32.8818, -15.5029) -> (30.142, -14.2481)
  line L161 (30.142, -14.2481) -> (30.4629, -13.5475)
  line L162 (30.4629, -13.5475) -> (32.8703, -14.6501)
  spline S183 degree 2 poles (32.8703, -14.6501) (33.1578, -14.7817) (33.6679, -14.961) (33.8355, -14.9509) knots 0 0 0 1 2 2 2
  spline S184 degree 2 poles (33.8355, -14.9509) (34.0167, -14.9469) (34.2859, -14.7388) (34.3949, -14.5007) knots 0 0 0 1 2 2 2
  spline S185 degree 2 poles (34.3949, -14.5007) (34.4977, -14.2761) (34.4431, -13.648) (34.33, -13.3137) knots 0 0 0 1 2 2 2
  line L163 (34.33, -13.3137) -> (31.222, -11.8902)
  line L164 (31.222, -11.8902) -> (31.5429, -11.1895)
  line L165 (31.5429, -11.1895) -> (35.7019, -13.0944)
  line L166 (35.7019, -13.0944) -> (35.381, -13.795)
  line L167 (35.381, -13.795) -> (34.9229, -13.5852)
  spline S186 degree 2 poles (34.9229, -13.5852) (35.0714, -13.9847) (35.1254, -14.6614) (34.9773, -14.9848) knots 0 0 0 1 2 2 2
  spline S187 degree 2 poles (34.9773, -14.9848) (34.8087, -15.3531) (34.2105, -15.7692) (33.7609, -15.7426) knots 0 0 0 1 2 2 2
  spline S188 degree 2 poles (33.7609, -15.7426) (33.9697, -16.224) (34.0578, -16.9925) (33.8974, -17.3428) knots 0 0 0 1 2 2 2
  spline S189 degree 2 poles (33.8974, -17.3428) (33.7739, -17.6123) (33.4062, -17.9763) (33.1435, -18.0516) knots 0 0 0 1 2 2 2
  spline S190 degree 2 poles (33.1435, -18.0516) (32.8787, -18.1314) (32.2285, -18.0563) (31.8018, -17.8609) knots 0 0 0 1 2 2 2
  line L168 (31.8018, -17.8609) -> (29.0621, -16.6061)
  line L169 (29.0621, -16.6061) -> (29.383, -15.9054)
  line L170 (27.6342, -18.6542) -> (28.1695, -17.8356)
  line L171 (28.1695, -17.8356) -> (29.1452, -18.4736)
  line L172 (29.1452, -18.4736) -> (28.6099, -19.2923)
  line L173 (28.6099, -19.2923) -> (27.6342, -18.6542)
  line L174 (30.487, -20.5197) -> (31.0223, -19.701)
  line L175 (31.0223, -19.701) -> (31.9981, -20.3391)
  line L176 (31.9981, -20.3391) -> (31.4628, -21.1577)
  line L177 (31.4628, -21.1577) -> (30.487, -20.5197)
  line L178 (22.7993, -24.3757) -> (24.8707, -22.2418)
  line L179 (24.8707, -22.2418) -> (25.3173, -22.6754)
  line L180 (25.3173, -22.6754) -> (24.5465, -23.4694)
  line L181 (24.5465, -23.4694) -> (27.478, -26.3149)
  line L182 (27.478, -26.3149) -> (28.2487, -25.5209)
  line L183 (28.2487, -25.5209) -> (28.6493, -25.9097)
  spline S191 degree 2 poles (28.6493, -25.9097) (28.2123, -26.3599) (28.0546, -27.033) (28.3816, -27.4054) knots 0 0 0 1 2 2 2
  line L184 (28.3816, -27.4054) -> (27.9411, -27.8592)
  line L185 (27.9411, -27.8592) -> (23.9995, -24.033)
  line L186 (23.9995, -24.033) -> (23.2459, -24.8093)
  line L187 (23.2459, -24.8093) -> (22.7993, -24.3757)
  line L188 (20.9433, -25.9423) -> (21.6953, -25.3169)
  line L189 (21.6953, -25.3169) -> (22.4408, -26.2133)
  line L190 (22.4408, -26.2133) -> (21.6887, -26.8387)
  line L191 (21.6887, -26.8387) -> (20.9433, -25.9423)
  spline S192 degree 2 poles (17.9987, -30.393) (17.7551, -30.027) (17.5736, -29.2458) (17.6342, -28.8732) knots 0 0 0 1 2 2 2
  spline S193 degree 2 poles (17.6342, -28.8732) (17.6948, -28.5006) (18.1544, -27.8091) (18.5492, -27.5464) knots 0 0 0 1 2 2 2
  spline S194 degree 2 poles (18.5492, -27.5464) (18.9111, -27.3055) (19.7252, -26.9952) (20.0692, -26.9503) knots 0 0 0 1 2 2 2
  line L192 (20.0692, -26.9503) -> (20.5481, -27.67)
  line L193 (20.5481, -27.67) -> (20.4987, -27.7029)
  spline S195 degree 2 poles (20.4987, -27.7029) (20.3823, -27.6973) (19.9918, -27.7435) (19.7711, -27.7954) knots 0 0 0 1 2 2 2
  spline S196 degree 2 poles (19.7711, -27.7954) (19.5231, -27.8596) (19.138, -28.0031) (18.9282, -28.1427) knots 0 0 0 1 2 2 2
  spline S197 degree 2 poles (18.9282, -28.1427) (18.7226, -28.2795) (18.4345, -28.6848) (18.4014, -28.9383) knots 0 0 0 1 2 2 2
  spline S198 degree 2 poles (18.4014, -28.9383) (18.3751, -29.1753) (18.5117, -29.6659) (18.6924, -29.9373) knots 0 0 0 1 2 2 2
  spline S199 degree 2 poles (18.6924, -29.9373) (18.873, -30.2088) (19.2509, -30.4557) (19.4674, -30.4778) knots 0 0 0 1 2 2 2
  spline S200 degree 2 poles (19.4674, -30.4778) (19.6962, -30.5096) (20.195, -30.3319) (20.4541, -30.1595) knots 0 0 0 1 2 2 2
  spline S201 degree 2 poles (20.4541, -30.1595) (20.7338, -29.9734) (21.2316, -29.5176) (21.3755, -29.3683) knots 0 0 0 1 2 2 2
  line L194 (21.3755, -29.3683) -> (23.1161, -31.984)
  line L195 (23.1161, -31.984) -> (20.3317, -33.8368)
  line L196 (20.3317, -33.8368) -> (19.9349, -33.2404)
  line L197 (19.9349, -33.2404) -> (22.0653, -31.8228)
  line L198 (22.0653, -31.8228) -> (21.165, -30.4697)
  spline S202 degree 2 poles (21.165, -30.4697) (21.0525, -30.5683) (20.8222, -30.7393) (20.7235, -30.805) knots 0 0 0 1 2 2 2
  spline S203 degree 2 poles (20.7235, -30.805) (20.3328, -31.065) (19.7092, -31.296) (19.3365, -31.271) knots 0 0 0 1 2 2 2
  spline S204 degree 2 poles (19.3365, -31.271) (18.9598, -31.2488) (18.3052, -30.8536) (17.9987, -30.393) knots 0 0 0 1 2 2 2
  line L199 (13.6633, -30.4583) -> (15.8661, -36.1424)
  line L200 (15.8661, -36.1424) -> (12.3101, -37.5205)
  line L201 (12.3101, -37.5205) -> (12.0495, -36.848)
  line L202 (12.0495, -36.848) -> (14.8501, -35.7626)
  line L203 (14.8501, -35.7626) -> (14.2467, -34.2057)
  line L204 (14.2467, -34.2057) -> (11.635, -35.2179)
  line L205 (11.635, -35.2179) -> (11.3744, -34.5454)
  line L206 (11.3744, -34.5454) -> (13.9861, -33.5332)
  line L207 (13.9861, -33.5332) -> (13.1685, -31.4236)
  line L208 (13.1685, -31.4236) -> (10.368, -32.5089)
  line L209 (10.368, -32.5089) -> (10.1073, -31.8364)
  line L210 (10.1073, -31.8364) -> (13.6633, -30.4583)
  line L211 (5.8535, -32.8826) -> (6.7707, -32.661)
  line L212 (6.7707, -32.661) -> (8.2549, -34.0709)
  line L213 (8.2549, -34.0709) -> (8.9603, -32.1318)
  line L214 (8.9603, -32.1318) -> (9.8102, -31.9263)
  line L215 (9.8102, -31.9263) -> (8.8015, -34.5029)
  line L216 (8.8015, -34.5029) -> (10.8704, -36.3763)
  line L217 (10.8704, -36.3763) -> (9.9533, -36.5979)
  line L218 (9.9533, -36.5979) -> (8.4773, -35.2013)
  line L219 (8.4773, -35.2013) -> (7.7781, -37.1237)
  line L220 (7.7781, -37.1237) -> (6.9282, -37.3291)
  line L221 (6.9282, -37.3291) -> (7.9296, -34.7645)
  line L222 (7.9296, -34.7645) -> (5.8535, -32.8826)
  spline S205 degree 2 poles (-2.1657, -36.4077) (-2.1752, -35.5728) (-1.5138, -34.2215) (-0.95, -33.8396) knots 0 0 0 1 2 2 2
  spline S206 degree 2 poles (-0.95, -33.8396) (-0.489, -33.5429) (0.4621, -33.3344) (1.203, -33.3259) knots 0 0 0 1 2 2 2
  line L223 (1.203, -33.3259) -> (2.6059, -33.3099)
  line L224 (2.6059, -33.3099) -> (2.6755, -39.4055)
  line L225 (2.6755, -39.4055) -> (1.2875, -39.4214)
  spline S207 degree 2 poles (1.2875, -39.4214) (0.428, -39.4312) (-0.553, -39.1855) (-0.9014, -38.9622) knots 0 0 0 1 2 2 2
  spline S208 degree 2 poles (-0.9014, -38.9622) (-1.4937, -38.5787) (-2.1555, -37.2968) (-2.1657, -36.4077) knots 0 0 0 1 2 2 2
  spline S209 degree 2 poles (-1.3209, -36.4079) (-1.3129, -37.1093) (-0.8372, -38.0969) (-0.3746, -38.3732) knots 0 0 0 1 2 2 2
  spline S210 degree 2 poles (-0.3746, -38.3732) (-0.0464, -38.5622) (0.6916, -38.7266) (1.2399, -38.7204) knots 0 0 0 1 2 2 2
  line L226 (1.2399, -38.7204) -> (1.8574, -38.7133)
  line L227 (1.8574, -38.7133) -> (1.8038, -34.0206)
  line L228 (1.8038, -34.0206) -> (1.1864, -34.0277)
  spline S211 degree 2 poles (1.1864, -34.0277) (0.6479, -34.0338) (-0.1651, -34.216) (-0.4935, -34.4519) knots 0 0 0 1 2 2 2
  spline S212 degree 2 poles (-0.4935, -34.4519) (-0.915, -34.7433) (-1.329, -35.6966) (-1.3209, -36.4079) knots 0 0 0 1 2 2 2
  line L229 (-3.791, -33.1235) -> (-3.0244, -33.2023)
  line L230 (-3.0244, -33.2023) -> (-3.492, -37.7528)
  line L231 (-3.492, -37.7528) -> (-4.2586, -37.674)
  line L232 (-4.2586, -37.674) -> (-3.791, -33.1235)
  line L233 (-4.3904, -38.4252) -> (-3.5206, -38.5146)
  line L234 (-3.5206, -38.5146) -> (-3.6024, -39.3107)
  line L235 (-3.6024, -39.3107) -> (-4.4722, -39.2213)
  line L236 (-4.4722, -39.2213) -> (-4.3904, -38.4252)
  spline S213 degree 2 poles (-7.5106, -32.9896) (-7.4051, -32.9402) (-7.0466, -32.7598) (-6.8868, -32.7162) knots 0 0 0 1 2 2 2
  spline S214 degree 2 poles (-6.8868, -32.7162) (-6.6669, -32.6493) (-6.2716, -32.6123) (-5.9325, -32.68) knots 0 0 0 1 2 2 2
  spline S215 degree 2 poles (-5.9325, -32.68) (-5.6564, -32.7351) (-5.199, -33.0431) (-5.0478, -33.2697) knots 0 0 0 1 2 2 2
  spline S216 degree 2 poles (-5.0478, -33.2697) (-4.9053, -33.4896) (-4.7956, -34.0757) (-4.8556, -34.3761) knots 0 0 0 1 2 2 2
  spline S217 degree 2 poles (-4.8556, -34.3761) (-4.9484, -34.8411) (-5.4724, -35.4216) (-5.9364, -35.5254) knots 0 0 0 1 2 2 2
  spline S218 degree 2 poles (-5.9364, -35.5254) (-6.3491, -35.6244) (-7.4022, -35.5502) (-8.0049, -35.4651) knots 0 0 0 1 2 2 2
  line L237 (-8.0049, -35.4651) -> (-8.0339, -35.6104)
  spline S219 degree 2 poles (-8.0339, -35.6104) (-8.0861, -35.872) (-7.991, -36.2285) (-7.8641, -36.3496) knots 0 0 0 1 2 2 2
  spline S220 degree 2 poles (-7.8641, -36.3496) (-7.7371, -36.4707) (-7.3321, -36.612) (-7.1093, -36.6565) knots 0 0 0 1 2 2 2
  spline S221 degree 2 poles (-7.1093, -36.6565) (-6.8477, -36.7087) (-6.1094, -36.6949) (-5.7258, -36.6153) knots 0 0 0 1 2 2 2
  line L238 (-5.7258, -36.6153) -> (-5.6822, -36.624)
  line L239 (-5.6822, -36.624) -> (-5.836, -37.3943)
  spline S222 degree 2 poles (-5.836, -37.3943) (-6.0559, -37.4108) (-6.8649, -37.4004) (-7.2476, -37.324) knots 0 0 0 1 2 2 2
  spline S223 degree 2 poles (-7.2476, -37.324) (-7.7126, -37.2312) (-8.3182, -36.9591) (-8.5324, -36.7199) knots 0 0 0 1 2 2 2
  spline S224 degree 2 poles (-8.5324, -36.7199) (-8.7428, -36.4865) (-8.8679, -35.852) (-8.7838, -35.4305) knots 0 0 0 1 2 2 2
  line L240 (-8.7838, -35.4305) -> (-8.1716, -32.364)
  line L241 (-8.1716, -32.364) -> (-7.4159, -32.5149)
  line L242 (-7.4159, -32.5149) -> (-7.5106, -32.9896)
  line L243 (-7.6364, -33.6194) -> (-7.8849, -34.8644)
  spline S225 degree 2 poles (-7.8849, -34.8644) (-7.6088, -34.8943) (-6.7737, -34.9754) (-6.5014, -34.9492) knots 0 0 0 1 2 2 2
  spline S226 degree 2 poles (-6.5014, -34.9492) (-6.1827, -34.9171) (-5.7139, -34.6127) (-5.6462, -34.2736) knots 0 0 0 1 2 2 2
  spline S227 degree 2 poles (-5.6462, -34.2736) (-5.5688, -33.8861) (-5.9265, -33.4066) (-6.3431, -33.3235) knots 0 0 0 1 2 2 2
  spline S228 degree 2 poles (-6.3431, -33.3235) (-6.6967, -33.2529) (-7.339, -33.442) (-7.6364, -33.6194) knots 0 0 0 1 2 2 2
  line L244 (-14.0747, -30.3026) -> (-15.0276, -32.773)
  spline S229 degree 2 poles (-15.0276, -32.773) (-15.1414, -33.068) (-15.2891, -33.5881) (-15.2687, -33.7548) knots 0 0 0 1 2 2 2
  spline S230 degree 2 poles (-15.2687, -33.7548) (-15.2537, -33.9354) (-15.0294, -34.1913) (-14.7851, -34.2856) knots 0 0 0 1 2 2 2
  spline S231 degree 2 poles (-14.7851, -34.2856) (-14.5639, -34.3709) (-13.952, -34.2945) (-13.5851, -34.1396) knots 0 0 0 1 2 2 2
  spline S232 degree 2 poles (-13.5851, -34.1396) (-13.5648, -34.0733) (-13.5047, -33.8899) (-13.4585, -33.7701) knots 0 0 0 1 2 2 2
  line L245 (-13.4585, -33.7701) -> (-12.3739, -30.9586)
  line L246 (-12.3739, -30.9586) -> (-11.6549, -31.236)
  line L247 (-11.6549, -31.236) -> (-12.6079, -33.7064)
  spline S233 degree 2 poles (-12.6079, -33.7064) (-12.7217, -34.0014) (-12.8694, -34.5215) (-12.849, -34.6883) knots 0 0 0 1 2 2 2
  spline S234 degree 2 poles (-12.849, -34.6883) (-12.8339, -34.8688) (-12.6097, -35.1247) (-12.3654, -35.219) knots 0 0 0 1 2 2 2
  spline S235 degree 2 poles (-12.3654, -35.219) (-12.1349, -35.3079) (-11.5113, -35.2149) (-11.1846, -35.0815) knots 0 0 0 1 2 2 2
  line L248 (-11.1846, -35.0815) -> (-9.9542, -31.892)
  line L249 (-9.9542, -31.892) -> (-9.2352, -32.1694)
  line L250 (-9.2352, -32.1694) -> (-10.8816, -36.4373)
  line L251 (-10.8816, -36.4373) -> (-11.6006, -36.16)
  line L252 (-11.6006, -36.16) -> (-11.4192, -35.6899)
  spline S236 degree 2 poles (-11.4192, -35.6899) (-11.8088, -35.8626) (-12.481, -35.958) (-12.8129, -35.83) knots 0 0 0 1 2 2 2
  spline S237 degree 2 poles (-12.8129, -35.83) (-13.1908, -35.6842) (-13.6428, -35.1127) (-13.6438, -34.6623) knots 0 0 0 1 2 2 2
  spline S238 degree 2 poles (-13.6438, -34.6623) (-14.1115, -34.9002) (-14.8731, -35.0353) (-15.2326, -34.8966) knots 0 0 0 1 2 2 2
  spline S239 degree 2 poles (-15.2326, -34.8966) (-15.5092, -34.7899) (-15.8951, -34.4451) (-15.9863, -34.1875) knots 0 0 0 1 2 2 2
  spline S240 degree 2 poles (-15.9863, -34.1875) (-16.0822, -33.9282) (-16.0471, -33.2746) (-15.8782, -32.8367) knots 0 0 0 1 2 2 2
  line L253 (-15.8782, -32.8367) -> (-14.7937, -30.0252)
  line L254 (-14.7937, -30.0252) -> (-14.0747, -30.3026)
  line L255 (-18.6126, -31.6874) -> (-17.7627, -32.1715)
  line L256 (-17.7627, -32.1715) -> (-18.3397, -33.1845)
  line L257 (-18.3397, -33.1845) -> (-19.1896, -32.7004)
  line L258 (-19.1896, -32.7004) -> (-18.6126, -31.6874)
  line L259 (-16.9255, -28.7255) -> (-16.0755, -29.2097)
  line L260 (-16.0755, -29.2097) -> (-16.6526, -30.2227)
  line L261 (-16.6526, -30.2227) -> (-17.5025, -29.7386)
  line L262 (-17.5025, -29.7386) -> (-16.9255, -28.7255)
  spline S241 degree 2 poles (-25.1539, -29.6154) (-24.9852, -29.7601) (-24.5808, -29.964) (-24.3649, -30.0386) knots 0 0 0 1 2 2 2
  spline S242 degree 2 poles (-24.3649, -30.0386) (-24.1603, -30.1035) (-23.8233, -30.1584) (-23.6856, -30.1724) knots 0 0 0 1 2 2 2
  line L263 (-23.6856, -30.1724) -> (-23.6481, -30.2046)
  line L264 (-23.6481, -30.2046) -> (-24.2111, -30.8606)
  spline S243 degree 2 poles (-24.2111, -30.8606) (-24.5068, -30.7956) (-25.3515, -30.3767) (-25.6627, -30.1096) knots 0 0 0 1 2 2 2
  spline S244 degree 2 poles (-25.6627, -30.1096) (-25.9776, -29.8394) (-26.3368, -29.3098) (-26.4122, -29.0108) knots 0 0 0 1 2 2 2
  spline S245 degree 2 poles (-26.4122, -29.0108) (-26.4892, -28.6908) (-26.3356, -28.0871) (-26.0911, -27.8021) knots 0 0 0 1 2 2 2
  spline S246 degree 2 poles (-26.0911, -27.8021) (-25.763, -27.4198) (-24.7652, -27.2735) (-24.3484, -27.501) knots 0 0 0 1 2 2 2
  line L265 (-24.3484, -27.501) -> (-24.3098, -27.456)
  spline S247 degree 2 poles (-24.3098, -27.456) (-24.4303, -27.3005) (-24.6481, -26.8792) (-24.6748, -26.622) knots 0 0 0 1 2 2 2
  spline S248 degree 2 poles (-24.6748, -26.622) (-24.7046, -26.3686) (-24.5243, -25.7943) (-24.2637, -25.4906) knots 0 0 0 1 2 2 2